Autodesk Fusion 360 part; units mm, degrees
(part 3 of 3)
sketch "M3 heat-set insert envelope sketch (1)" plane through (0, 0, 52) normal (0, 0, 1) x (1, 0, 0) in component "19 Rear M3 fastener envelopes TBD"
  circle A0 centre (-40, 90) radius 2.1
  dimension "d1035" = 40
  dimension "d1036" = 90
  dimension "d1037" = 2.1
  measures "d1035" horizontal distance of origin A0.centre
  measures "d1036" vertical distance of origin A0.centre
  measures "d1037" radius of A0
extrude "M3 heat-set insert envelope (1)" add sketch "M3 heat-set insert envelope sketch (1)" along normal blind 5 separate body makes body 40 in component "19 Rear M3 fastener envelopes TBD"
ref_plane "WorkPlane6" through (0, 0, 52) normal (0, 0, 1) x (1, 0, 0) in component "19 Rear M3 fastener envelopes TBD"
sketch "Insert thread clearance envelope sketch (1)" plane through (0, 0, 52) normal (0, 0, 1) x (1, 0, 0) in component "19 Rear M3 fastener envelopes TBD"
  circle A0 centre (-40, 90) radius 1.55
  dimension "d1042" = 40
  dimension "d1043" = 90
  dimension "d1044" = 1.55
  measures "d1042" horizontal distance of origin A0.centre
  measures "d1043" vertical distance of origin A0.centre
  measures "d1044" radius of A0
extrude "Insert thread clearance envelope (1)" cut sketch "Insert thread clearance envelope sketch (1)" along normal blind 5 bodies 40 in component "19 Rear M3 fastener envelopes TBD"
ref_plane "WorkPlane7" through (0, 0, 54.2) normal (0, 0, 1) x (1, 0, 0) in component "19 Rear M3 fastener envelopes TBD"
sketch "M3 screw shaft envelope sketch (1)" plane through (0, 0, 54.2) normal (0, 0, 1) x (1, 0, 0) in component "19 Rear M3 fastener envelopes TBD"
  circle A0 centre (-40, 90) radius 1.45
  dimension "d1049" = 40
  dimension "d1050" = 90
  dimension "d1051" = 1.45
  measures "d1049" horizontal distance of origin A0.centre
  measures "d1050" vertical distance of origin A0.centre
  measures "d1051" radius of A0
extrude "M3 screw shaft envelope (1)" add sketch "M3 screw shaft envelope sketch (1)" along normal blind 4 separate body makes body 41 in component "19 Rear M3 fastener envelopes TBD"
ref_plane "WorkPlane8" through (0, 0, 58.2) normal (0, 0, 1) x (1, 0, 0) in component "19 Rear M3 fastener envelopes TBD"
sketch "M3 low head envelope sketch (1)" plane through (0, 0, 58.2) normal (0, 0, 1) x (1, 0, 0) in component "19 Rear M3 fastener envelopes TBD"
  circle A0 centre (-40, 90) radius 2.75
  dimension "d1056" = 40
  dimension "d1057" = 90
  dimension "d1058" = 2.75
  measures "d1056" horizontal distance of origin A0.centre
  measures "d1057" vertical distance of origin A0.centre
  measures "d1058" radius of A0
extrude "M3 low head envelope (1)" add sketch "M3 low head envelope sketch (1)" along normal blind 1.8 separate body makes body 42 in component "19 Rear M3 fastener envelopes TBD"
ref_plane "WorkPlane10" through (0, 0, 58.2) normal (0, 0, 1) x (1, 0, 0) in component "02 Single rear cover"
sketch "M3 head recess sketch (2)" plane through (0, 0, 58.2) normal (0, 0, 1) x (1, 0, 0) in component "02 Single rear cover"
  circle A0 centre (-40, 172) radius 3
  dimension "d1063" = 40
  dimension "d1064" = 172
  dimension "d1065" = 3
  measures "d1063" horizontal distance of origin A0.centre
  measures "d1064" vertical distance of origin A0.centre
  measures "d1065" radius of A0
extrude "M3 head recess (2)" cut sketch "M3 head recess sketch (2)" along normal blind 1.9 bodies 2 in component "02 Single rear cover"
ref_plane "WorkPlane9" through (0, 0, 52) normal (0, 0, 1) x (1, 0, 0) in component "19 Rear M3 fastener envelopes TBD"
sketch "M3 heat-set insert envelope sketch (2)" plane through (0, 0, 52) normal (0, 0, 1) x (1, 0, 0) in component "19 Rear M3 fastener envelopes TBD"
  circle A0 centre (-40, 172) radius 2.1
  dimension "d1070" = 40
  dimension "d1071" = 172
  dimension "d1072" = 2.1
  measures "d1070" horizontal distance of origin A0.centre
  measures "d1071" vertical distance of origin A0.centre
  measures "d1072" radius of A0
extrude "M3 heat-set insert envelope (2)" add sketch "M3 heat-set insert envelope sketch (2)" along normal blind 5 separate body makes body 43 in component "19 Rear M3 fastener envelopes TBD"
ref_plane "WorkPlane10" through (0, 0, 52) normal (0, 0, 1) x (1, 0, 0) in component "19 Rear M3 fastener envelopes TBD"
sketch "Insert thread clearance envelope sketch (2)" plane through (0, 0, 52) normal (0, 0, 1) x (1, 0, 0) in component "19 Rear M3 fastener envelopes TBD"
  circle A0 centre (-40, 172) radius 1.55
  dimension "d1077" = 40
  dimension "d1078" = 172
  dimension "d1079" = 1.55
  measures "d1077" horizontal distance of origin A0.centre
  measures "d1078" vertical distance of origin A0.centre
  measures "d1079" radius of A0
extrude "Insert thread clearance envelope (2)" cut sketch "Insert thread clearance envelope sketch (2)" along normal blind 5 bodies 43 in component "19 Rear M3 fastener envelopes TBD"
ref_plane "WorkPlane11" through (0, 0, 54.2) normal (0, 0, 1) x (1, 0, 0) in component "19 Rear M3 fastener envelopes TBD"
sketch "M3 screw shaft envelope sketch (2)" plane through (0, 0, 54.2) normal (0, 0, 1) x (1, 0, 0) in component "19 Rear M3 fastener envelopes TBD"
  circle A0 centre (-40, 172) radius 1.45
  dimension "d1084" = 40
  dimension "d1085" = 172
  dimension "d1086" = 1.45
  measures "d1084" horizontal distance of origin A0.centre
  measures "d1085" vertical distance of origin A0.centre
  measures "d1086" radius of A0
extrude "M3 screw shaft envelope (2)" add sketch "M3 screw shaft envelope sketch (2)" along normal blind 4 separate body makes body 44 in component "19 Rear M3 fastener envelopes TBD"
ref_plane "WorkPlane12" through (0, 0, 58.2) normal (0, 0, 1) x (1, 0, 0) in component "19 Rear M3 fastener envelopes TBD"
sketch "M3 low head envelope sketch (2)" plane through (0, 0, 58.2) normal (0, 0, 1) x (1, 0, 0) in component "19 Rear M3 fastener envelopes TBD"
  circle A0 centre (-40, 172) radius 2.75
  dimension "d1091" = 40
  dimension "d1092" = 172
  dimension "d1093" = 2.75
  measures "d1091" horizontal distance of origin A0.centre
  measures "d1092" vertical distance of origin A0.centre
  measures "d1093" radius of A0
extrude "M3 low head envelope (2)" add sketch "M3 low head envelope sketch (2)" along normal blind 1.8 separate body makes body 45 in component "19 Rear M3 fastener envelopes TBD"
ref_plane "WorkPlane11" through (0, 0, 58.2) normal (0, 0, 1) x (1, 0, 0) in component "02 Single rear cover"
sketch "M3 head recess sketch (3)" plane through (0, 0, 58.2) normal (0, 0, 1) x (1, 0, 0) in component "02 Single rear cover"
  circle A0 centre (40, 8) radius 3
  dimension "d1098" = 40
  dimension "d1099" = 8
  dimension "d1100" = 3
  measures "d1098" horizontal distance of origin A0.centre
  measures "d1099" vertical distance of origin A0.centre
  measures "d1100" radius of A0
extrude "M3 head recess (3)" cut sketch "M3 head recess sketch (3)" along normal blind 1.9 bodies 2 in component "02 Single rear cover"
ref_plane "WorkPlane13" through (0, 0, 52) normal (0, 0, 1) x (1, 0, 0) in component "19 Rear M3 fastener envelopes TBD"
sketch "M3 heat-set insert envelope sketch (3)" plane through (0, 0, 52) normal (0, 0, 1) x (1, 0, 0) in component "19 Rear M3 fastener envelopes TBD"
  circle A0 centre (40, 8) radius 2.1
  dimension "d1105" = 40
  dimension "d1106" = 8
  dimension "d1107" = 2.1
  measures "d1105" horizontal distance of origin A0.centre
  measures "d1106" vertical distance of origin A0.centre
  measures "d1107" radius of A0
extrude "M3 heat-set insert envelope (3)" add sketch "M3 heat-set insert envelope sketch (3)" along normal blind 5 separate body makes body 46 in component "19 Rear M3 fastener envelopes TBD"
ref_plane "WorkPlane14" through (0, 0, 52) normal (0, 0, 1) x (1, 0, 0) in component "19 Rear M3 fastener envelopes TBD"
sketch "Insert thread clearance envelope sketch (3)" plane through (0, 0, 52) normal (0, 0, 1) x (1, 0, 0) in component "19 Rear M3 fastener envelopes TBD"
  circle A0 centre (40, 8) radius 1.55
  dimension "d1112" = 40
  dimension "d1113" = 8
  dimension "d1114" = 1.55
  measures "d1112" horizontal distance of origin A0.centre
  measures "d1113" vertical distance of origin A0.centre
  measures "d1114" radius of A0
extrude "Insert thread clearance envelope (3)" cut sketch "Insert thread clearance envelope sketch (3)" along normal blind 5 bodies 46 in component "19 Rear M3 fastener envelopes TBD"
ref_plane "WorkPlane15" through (0, 0, 54.2) normal (0, 0, 1) x (1, 0, 0) in component "19 Rear M3 fastener envelopes TBD"
sketch "M3 screw shaft envelope sketch (3)" plane through (0, 0, 54.2) normal (0, 0, 1) x (1, 0, 0) in component "19 Rear M3 fastener envelopes TBD"
  circle A0 centre (40, 8) radius 1.45
  dimension "d1119" = 40
  dimension "d1120" = 8
  dimension "d1121" = 1.45
  measures "d1119" horizontal distance of origin A0.centre
  measures "d1120" vertical distance of origin A0.centre
  measures "d1121" radius of A0
extrude "M3 screw shaft envelope (3)" add sketch "M3 screw shaft envelope sketch (3)" along normal blind 4 separate body makes body 47 in component "19 Rear M3 fastener envelopes TBD"
ref_plane "WorkPlane16" through (0, 0, 58.2) normal (0, 0, 1) x (1, 0, 0) in component "19 Rear M3 fastener envelopes TBD"
sketch "M3 low head envelope sketch (3)" plane through (0, 0, 58.2) normal (0, 0, 1) x (1, 0, 0) in component "19 Rear M3 fastener envelopes TBD"
  circle A0 centre (40, 8) radius 2.75
  dimension "d1126" = 40
  dimension "d1127" = 8
  dimension "d1128" = 2.75
  measures "d1126" horizontal distance of origin A0.centre
  measures "d1127" vertical distance of origin A0.centre
  measures "d1128" radius of A0
extrude "M3 low head envelope (3)" add sketch "M3 low head envelope sketch (3)" along normal blind 1.8 separate body makes body 48 in component "19 Rear M3 fastener envelopes TBD"
ref_plane "WorkPlane12" through (0, 0, 58.2) normal (0, 0, 1) x (1, 0, 0) in component "02 Single rear cover"
sketch "M3 head recess sketch (4)" plane through (0, 0, 58.2) normal (0, 0, 1) x (1, 0, 0) in component "02 Single rear cover"
  circle A0 centre (40, 90) radius 3
  dimension "d1133" = 40
  dimension "d1134" = 90
  dimension "d1135" = 3
  measures "d1133" horizontal distance of origin A0.centre
  measures "d1134" vertical distance of origin A0.centre
  measures "d1135" radius of A0
extrude "M3 head recess (4)" cut sketch "M3 head recess sketch (4)" along normal blind 1.9 bodies 2 in component "02 Single rear cover"
ref_plane "WorkPlane17" through (0, 0, 52) normal (0, 0, 1) x (1, 0, 0) in component "19 Rear M3 fastener envelopes TBD"
sketch "M3 heat-set insert envelope sketch (4)" plane through (0, 0, 52) normal (0, 0, 1) x (1, 0, 0) in component "19 Rear M3 fastener envelopes TBD"
  circle A0 centre (40, 90) radius 2.1
  dimension "d1140" = 40
  dimension "d1141" = 90
  dimension "d1142" = 2.1
  measures "d1140" horizontal distance of origin A0.centre
  measures "d1141" vertical distance of origin A0.centre
  measures "d1142" radius of A0
extrude "M3 heat-set insert envelope (4)" add sketch "M3 heat-set insert envelope sketch (4)" along normal blind 5 separate body makes body 49 in component "19 Rear M3 fastener envelopes TBD"
ref_plane "WorkPlane18" through (0, 0, 52) normal (0, 0, 1) x (1, 0, 0) in component "19 Rear M3 fastener envelopes TBD"
sketch "Insert thread clearance envelope sketch (4)" plane through (0, 0, 52) normal (0, 0, 1) x (1, 0, 0) in component "19 Rear M3 fastener envelopes TBD"
  circle A0 centre (40, 90) radius 1.55
  dimension "d1147" = 40
  dimension "d1148" = 90
  dimension "d1149" = 1.55
  measures "d1147" horizontal distance of origin A0.centre
  measures "d1148" vertical distance of origin A0.centre
  measures "d1149" radius of A0
extrude "Insert thread clearance envelope (4)" cut sketch "Insert thread clearance envelope sketch (4)" along normal blind 5 bodies 49 in component "19 Rear M3 fastener envelopes TBD"
ref_plane "WorkPlane19" through (0, 0, 54.2) normal (0, 0, 1) x (1, 0, 0) in component "19 Rear M3 fastener envelopes TBD"
sketch "M3 screw shaft envelope sketch (4)" plane through (0, 0, 54.2) normal (0, 0, 1) x (1, 0, 0) in component "19 Rear M3 fastener envelopes TBD"
  circle A0 centre (40, 90) radius 1.45
  dimension "d1154" = 40
  dimension "d1155" = 90
  dimension "d1156" = 1.45
  measures "d1154" horizontal distance of origin A0.centre
  measures "d1155" vertical distance of origin A0.centre
  measures "d1156" radius of A0
extrude "M3 screw shaft envelope (4)" add sketch "M3 screw shaft envelope sketch (4)" along normal blind 4 separate body makes body 50 in component "19 Rear M3 fastener envelopes TBD"
ref_plane "WorkPlane20" through (0, 0, 58.2) normal (0, 0, 1) x (1, 0, 0) in component "19 Rear M3 fastener envelopes TBD"
sketch "M3 low head envelope sketch (4)" plane through (0, 0, 58.2) normal (0, 0, 1) x (1, 0, 0) in component "19 Rear M3 fastener envelopes TBD"
  circle A0 centre (40, 90) radius 2.75
  dimension "d1161" = 40
  dimension "d1162" = 90
  dimension "d1163" = 2.75
  measures "d1161" horizontal distance of origin A0.centre
  measures "d1162" vertical distance of origin A0.centre
  measures "d1163" radius of A0
extrude "M3 low head envelope (4)" add sketch "M3 low head envelope sketch (4)" along normal blind 1.8 separate body makes body 51 in component "19 Rear M3 fastener envelopes TBD"
ref_plane "WorkPlane13" through (0, 0, 58.2) normal (0, 0, 1) x (1, 0, 0) in component "02 Single rear cover"
sketch "M3 head recess sketch (5)" plane through (0, 0, 58.2) normal (0, 0, 1) x (1, 0, 0) in component "02 Single rear cover"
  circle A0 centre (40, 172) radius 3
  dimension "d1168" = 40
  dimension "d1169" = 172
  dimension "d1170" = 3
  measures "d1168" horizontal distance of origin A0.centre
  measures "d1169" vertical distance of origin A0.centre
  measures "d1170" radius of A0
extrude "M3 head recess (5)" cut sketch "M3 head recess sketch (5)" along normal blind 1.9 bodies 2 in component "02 Single rear cover"
ref_plane "WorkPlane21" through (0, 0, 52) normal (0, 0, 1) x (1, 0, 0) in component "19 Rear M3 fastener envelopes TBD"
sketch "M3 heat-set insert envelope sketch (5)" plane through (0, 0, 52) normal (0, 0, 1) x (1, 0, 0) in component "19 Rear M3 fastener envelopes TBD"
  circle A0 centre (40, 172) radius 2.1
  dimension "d1175" = 40
  dimension "d1176" = 172
  dimension "d1177" = 2.1
  measures "d1175" horizontal distance of origin A0.centre
  measures "d1176" vertical distance of origin A0.centre
  measures "d1177" radius of A0
extrude "M3 heat-set insert envelope (5)" add sketch "M3 heat-set insert envelope sketch (5)" along normal blind 5 separate body makes body 52 in component "19 Rear M3 fastener envelopes TBD"
ref_plane "WorkPlane22" through (0, 0, 52) normal (0, 0, 1) x (1, 0, 0) in component "19 Rear M3 fastener envelopes TBD"
sketch "Insert thread clearance envelope sketch (5)" plane through (0, 0, 52) normal (0, 0, 1) x (1, 0, 0) in component "19 Rear M3 fastener envelopes TBD"
  circle A0 centre (40, 172) radius 1.55
  dimension "d1182" = 40
  dimension "d1183" = 172
  dimension "d1184" = 1.55
  measures "d1182" horizontal distance of origin A0.centre
  measures "d1183" vertical distance of origin A0.centre
  measures "d1184" radius of A0
extrude "Insert thread clearance envelope (5)" cut sketch "Insert thread clearance envelope sketch (5)" along normal blind 5 bodies 52 in component "19 Rear M3 fastener envelopes TBD"
ref_plane "WorkPlane23" through (0, 0, 54.2) normal (0, 0, 1) x (1, 0, 0) in component "19 Rear M3 fastener envelopes TBD"
sketch "M3 screw shaft envelope sketch (5)" plane through (0, 0, 54.2) normal (0, 0, 1) x (1, 0, 0) in component "19 Rear M3 fastener envelopes TBD"
  circle A0 centre (40, 172) radius 1.45
  dimension "d1189" = 40
  dimension "d1190" = 172
  dimension "d1191" = 1.45
  measures "d1189" horizontal distance of origin A0.centre
  measures "d1190" vertical distance of origin A0.centre
  measures "d1191" radius of A0
extrude "M3 screw shaft envelope (5)" add sketch "M3 screw shaft envelope sketch (5)" along normal blind 4 separate body makes body 53 in component "19 Rear M3 fastener envelopes TBD"
ref_plane "WorkPlane24" through (0, 0, 58.2) normal (0, 0, 1) x (1, 0, 0) in component "19 Rear M3 fastener envelopes TBD"
sketch "M3 low head envelope sketch (5)" plane through (0, 0, 58.2) normal (0, 0, 1) x (1, 0, 0) in component "19 Rear M3 fastener envelopes TBD"
  circle A0 centre (40, 172) radius 2.75
  dimension "d1196" = 40
  dimension "d1197" = 172
  dimension "d1198" = 2.75
  measures "d1196" horizontal distance of origin A0.centre
  measures "d1197" vertical distance of origin A0.centre
  measures "d1198" radius of A0
extrude "M3 low head envelope (5)" add sketch "M3 low head envelope sketch (5)" along normal blind 1.8 separate body makes body 54 in component "19 Rear M3 fastener envelopes TBD"
component "01 Main housing" placed x (1, 0, 0) y (0, 1, 0) z (0, 0, 1) at (0, 0, 0)
component "02 Single rear cover" placed x (1, 0, 0) y (0, 1, 0) z (0, 0, 1) at (0, 0, 0)
component "03 Removable sampling chamber" placed x (1, 0, 0) y (0, 1, 0) z (0, 0, 1) at (0, 0, 0)
component "04 Internal chamber lid" placed x (1, 0, 0) y (0, 1, 0) z (0, 0, 1) at (0, 0, 0)
component "05 Feedthrough seal envelope TBD" placed x (1, 0, 0) y (0, 1, 0) z (0, 0, 1) at (0, 0, 0)
component "06 Gas fitting envelopes TBD" placed x (1, 0, 0) y (0, 1, 0) z (0, 0, 1) at (0, 0, 0)
component "07 Guition 4.3in envelope — depth TBD" placed x (1, 0, 0) y (0, 1, 0) z (0, 0, 1) at (0, 0, 0)
component "08 Active display reference" placed x (1, 0, 0) y (0, 1, 0) z (0, 0, 1) at (0, 0, 0)
component "09 Removable electronics carrier" placed x (1, 0, 0) y (0, 1, 0) z (0, 0, 1) at (0, 0, 0)
component "10 Future PCB and component envelope TBD" placed x (1, 0, 0) y (0, 1, 0) z (0, 0, 1) at (0, 0, 0)
component "11 Protected FMA holder envelope TBD" placed x (1, 0, 0) y (0, 1, 0) z (0, 0, 1) at (0, 0, 0)
component "12 Two 18650 cell envelopes" placed x (1, 0, 0) y (0, 1, 0) z (0, 0, 1) at (0, 0, 0)
component "13 Battery plug and cable clearance TBD" placed x (1, 0, 0) y (0, 1, 0) z (0, 0, 1) at (0, 0, 0)
component "14 Supported USB-C mounting insert TBD" placed x (1, 0, 0) y (0, 1, 0) z (0, 0, 1) at (0, 0, 0)
component "15 USB daughterboard envelope 0.60mm" placed x (1, 0, 0) y (0, 1, 0) z (0, 0, 1) at (0, 0, 0)
component "16 Right momentary button envelope TBD" placed x (1, 0, 0) y (0, 1, 0) z (0, 0, 1) at (0, 0, 0)
component "18 Wiring route clearance envelopes" placed x (1, 0, 0) y (0, 1, 0) z (0, 0, 1) at (0, 0, 0)
component "17 Chamber sensor envelopes TBD" placed x (1, 0, 0) y (0, 1, 0) z (0, 0, 1) at (0, 0, 0)
component "19 Rear M3 fastener envelopes TBD" placed x (1, 0, 0) y (0, 1, 0) z (0, 0, 1) at (0, 0, 0)
equation "CaseWidth = 95 mm" comment "Provisional outer width"
equation "CaseHeight = 180 mm" comment "Provisional outer height"
equation "CaseDepth = 60 mm" comment "Provisional total depth including rear cover"
equation "Wall = 3 mm" comment "Initial PLA shell wall"
equation "Cover = 3 mm" comment "Single rear cover thickness"
equation "CornerRadius = 8 mm" comment "Outside corner radius"
equation "CoverGap = 0.25 mm" comment "Provisional cover seating clearance"
equation "DisplayWidth = 69.41 mm" comment "Verified conservative Guition module outline"
equation "DisplayHeight = 117.01 mm" comment "Verified conservative Guition module outline"
equation "DisplayDepth = 13.8 mm" comment "PROVISIONAL: shell-variant depth; confirm purchased unit"
equation "DisplayBottom = 10 mm" comment "Module lower edge"
equation "ActiveWidth = 56.16 mm" comment "Verified active display width"
equation "ActiveHeight = 93.60 mm" comment "Verified active display height"
equation "WindowMargin = 0.5 mm" comment "Provisional margin around active area"
equation "BossInset = 7.5 mm" comment "Rear-cover screw centre inset from left/right"
equation "BossRadius = 4.5 mm" comment "Cover screw boss outer radius"
equation "InsertRadius = 2.1 mm" comment "PROVISIONAL M3 insert pilot radius; fit coupon required"
equation "InsertDepth = 5 mm" comment "PROVISIONAL M3 insert length"
equation "ScrewClearance = 1.7 mm" comment "M3 rear-cover clearance radius"
equation "ChamberWidth = 70 mm" comment "Removable chamber outside width"
equation "ChamberHeight = 43 mm" comment "Removable chamber outside height"
equation "ChamberTopGap = 5 mm" comment "Clearance to case top"
equation "ChamberBottom = CaseHeight - ChamberTopGap - ChamberHeight" comment "Derived chamber lower edge"
equation "ChamberFront = 3.5 mm" comment "Chamber front wall position"
equation "ChamberWall = 2 mm" comment "Concept chamber wall; seal details pending"
equation "ChamberLid = 2 mm" comment "Internally accessible chamber lid"
equation "ChamberRear = CaseDepth - Cover - 0.5 mm" comment "Rear of closed chamber"
equation "GasY = ChamberBottom + ChamberHeight / 2" comment "Gas inlet/outlet elevation"
equation "GasZ = 12 mm" comment "Gas path centre depth"
equation "GasBoreRadius = 2.5 mm" comment "5 mm nominal tube ID"
equation "GasPassRadius = 4.5 mm" comment "PROVISIONAL housing clearance for side fitting"
equation "UsbY = 68 mm" comment "Left charging connector centre height"
equation "UsbZ = 34 mm" comment "USB connector depth centre"
equation "ButtonY = 102 mm" comment "Right-side power button centre height"
equation "ButtonZ = 42 mm" comment "Button depth centre"
equation "ButtonRadius = 6 mm" comment "Owned nominal 12 mm mounting diameter; confirm"
equation "d42 = -( -CaseWidth / 2 )"
equation "d43 = CaseWidth"
equation "d44 = CaseHeight"
equation "d45 = CaseDepth - Cover"
equation "d48 = CornerRadius"
equation "d49 = Wall"
equation "d51 = -( -CaseWidth / 2 + Wall )"
equation "d52 = Wall"
equation "d53 = CaseWidth - 2 * Wall"
equation "d54 = CaseHeight - 2 * Wall"
equation "d55 = CaseDepth"
equation "d58 = CornerRadius - Wall"
equation "d61 = -( -( ActiveWidth + 2 * WindowMargin ) / 2 )"
equation "d62 = DisplayBottom + ( DisplayHeight - ActiveHeight ) / 2 - WindowMargin"
equation "d63 = ActiveWidth + 2 * WindowMargin"
equation "d64 = ActiveHeight + 2 * WindowMargin"
equation "d65 = Wall + 2 mm"
equation "d67 = Wall"
equation "d69 = -( -CaseWidth / 2 + BossInset )"
equation "d71 = BossRadius"
equation "d72 = CaseDepth - Cover - Wall"
equation "d74 = Wall"
equation "d76 = -( -CaseWidth / 2 + Wall )"
equation "d77 = ( 8 mm ) - BossRadius"
equation "d78 = BossInset - Wall"
equation "d79 = 2 * BossRadius"
equation "d80 = CaseDepth - Cover - Wall"
equation "d82 = CaseDepth - Cover - InsertDepth"
equation "d84 = -( -CaseWidth / 2 + BossInset )"
equation "d86 = InsertRadius"
equation "d87 = InsertDepth + 0.1 mm"
equation "d89 = Wall"
equation "d91 = -( -CaseWidth / 2 + BossInset )"
equation "d92 = CaseHeight / 2"
equation "d93 = BossRadius"
equation "d94 = CaseDepth - Cover - Wall"
equation "d96 = Wall"
equation "d98 = -( -CaseWidth / 2 + Wall )"
equation "d99 = ( CaseHeight / 2 ) - BossRadius"
equation "d100 = BossInset - Wall"
equation "d101 = 2 * BossRadius"
equation "d102 = CaseDepth - Cover - Wall"
equation "d104 = CaseDepth - Cover - InsertDepth"
equation "d106 = -( -CaseWidth / 2 + BossInset )"
equation "d107 = CaseHeight / 2"
equation "d108 = InsertRadius"
equation "d109 = InsertDepth + 0.1 mm"
equation "d111 = Wall"
equation "d113 = -( -CaseWidth / 2 + BossInset )"
equation "d114 = CaseHeight - 8 mm"
equation "d115 = BossRadius"
equation "d116 = CaseDepth - Cover - Wall"
equation "d118 = Wall"
equation "d120 = -( -CaseWidth / 2 + Wall )"
equation "d121 = ( CaseHeight - 8 mm ) - BossRadius"
equation "d122 = BossInset - Wall"
equation "d123 = 2 * BossRadius"
equation "d124 = CaseDepth - Cover - Wall"
equation "d126 = CaseDepth - Cover - InsertDepth"
equation "d128 = -( -CaseWidth / 2 + BossInset )"
equation "d129 = CaseHeight - 8 mm"
equation "d130 = InsertRadius"
equation "d131 = InsertDepth + 0.1 mm"
equation "d133 = Wall"
equation "d135 = CaseWidth / 2 - BossInset"
equation "d137 = BossRadius"
equation "d138 = CaseDepth - Cover - Wall"
equation "d140 = Wall"
equation "d142 = CaseWidth / 2 - BossInset"
equation "d143 = ( 8 mm ) - BossRadius"
equation "d144 = BossInset - Wall"
equation "d145 = 2 * BossRadius"
equation "d146 = CaseDepth - Cover - Wall"
equation "d148 = CaseDepth - Cover - InsertDepth"
equation "d150 = CaseWidth / 2 - BossInset"
equation "d152 = InsertRadius"
equation "d153 = InsertDepth + 0.1 mm"
equation "d155 = Wall"
equation "d157 = CaseWidth / 2 - BossInset"
equation "d158 = CaseHeight / 2"
equation "d159 = BossRadius"
equation "d160 = CaseDepth - Cover - Wall"
equation "d162 = Wall"
equation "d164 = CaseWidth / 2 - BossInset"
equation "d165 = ( CaseHeight / 2 ) - BossRadius"
equation "d166 = BossInset - Wall"
equation "d167 = 2 * BossRadius"
equation "d168 = CaseDepth - Cover - Wall"
equation "d170 = CaseDepth - Cover - InsertDepth"
equation "d172 = CaseWidth / 2 - BossInset"
equation "d173 = CaseHeight / 2"
equation "d174 = InsertRadius"
equation "d175 = InsertDepth + 0.1 mm"
equation "d177 = Wall"
equation "d179 = CaseWidth / 2 - BossInset"
equation "d180 = CaseHeight - 8 mm"
equation "d181 = BossRadius"
equation "d182 = CaseDepth - Cover - Wall"
equation "d184 = Wall"
equation "d186 = CaseWidth / 2 - BossInset"
equation "d187 = ( CaseHeight - 8 mm ) - BossRadius"
equation "d188 = BossInset - Wall"
equation "d189 = 2 * BossRadius"
equation "d190 = CaseDepth - Cover - Wall"
equation "d192 = CaseDepth - Cover - InsertDepth"
equation "d194 = CaseWidth / 2 - BossInset"
equation "d195 = CaseHeight - 8 mm"
equation "d196 = InsertRadius"
equation "d197 = InsertDepth + 0.1 mm"
equation "d199 = -CaseWidth / 2 - 1 mm"
equation "d201 = -( -( GasZ ) )"
equation "d202 = GasY"
equation "d203 = GasPassRadius"
equation "d204 = CaseWidth + 2 mm"
equation "d206 = -CaseWidth / 2 - 1 mm"
equation "d208 = -( -( ButtonZ ) )"
equation "d209 = ButtonY"
equation "d210 = ButtonRadius"
equation "d211 = Wall + 2 mm"
equation "d213 = CaseWidth / 2 - Wall - 1 mm"
equation "d215 = -( -( ( UsbZ - 8 mm ) + ( 16 mm ) ) )"
equation "d216 = UsbY - 10 mm"
equation "d219 = Wall + 2 mm"
equation "d221 = CaseDepth - Cover + CoverGap"
equation "d223 = -( -CaseWidth / 2 )"
equation "d224 = CaseWidth"
equation "d225 = CaseHeight"
equation "d226 = Cover - CoverGap"
equation "d229 = CornerRadius"
equation "d230 = CaseDepth - Cover"
equation "d232 = -( -CaseWidth / 2 + BossInset )"
equation "d234 = ScrewClearance"
equation "d235 = Cover + 1 mm"
equation "d237 = CaseDepth - Cover"
equation "d239 = -( -CaseWidth / 2 + BossInset )"
equation "d240 = CaseHeight / 2"
equation "d241 = ScrewClearance"
equation "d242 = Cover + 1 mm"
equation "d244 = CaseDepth - Cover"
equation "d246 = -( -CaseWidth / 2 + BossInset )"
equation "d247 = CaseHeight - 8 mm"
equation "d248 = ScrewClearance"
equation "d249 = Cover + 1 mm"
equation "d251 = CaseDepth - Cover"
equation "d253 = CaseWidth / 2 - BossInset"
equation "d255 = ScrewClearance"
equation "d256 = Cover + 1 mm"
equation "d258 = CaseDepth - Cover"
equation "d260 = CaseWidth / 2 - BossInset"
equation "d261 = CaseHeight / 2"
equation "d262 = ScrewClearance"
equation "d263 = Cover + 1 mm"
equation "d265 = CaseDepth - Cover"
equation "d267 = CaseWidth / 2 - BossInset"
equation "d268 = CaseHeight - 8 mm"
equation "d269 = ScrewClearance"
equation "d270 = Cover + 1 mm"
equation "d272 = ChamberFront"
equation "d274 = -( -ChamberWidth / 2 )"
equation "d275 = ChamberBottom"
equation "d276 = ChamberWidth"
equation "d277 = ChamberHeight"
equation "d278 = ChamberRear - ChamberFront - ChamberLid"
equation "d280 = ChamberFront + ChamberWall"
equation "d282 = -( -ChamberWidth / 2 + ChamberWall )"
equation "d283 = ChamberBottom + ChamberWall"
equation "d284 = ChamberWidth - 2 * ChamberWall"
equation "d285 = ChamberHeight - 2 * ChamberWall"
equation "d286 = ChamberRear - ChamberFront"
equation "d288 = -ChamberWidth / 2 - 1 mm"
equation "d290 = -( -( GasZ ) )"
equation "d291 = GasY"
equation "d293 = ChamberWidth + 2 mm"
equation "d295 = ChamberFront + ChamberWall"
equation "d297 = -( -ChamberWidth / 2 + 5 mm )"
equation "d298 = ChamberBottom + 4 mm"
equation "d300 = ChamberRear - ChamberLid - ChamberFront - ChamberWall"
equation "d302 = ChamberRear - ChamberLid - 4 mm"
equation "d304 = -( -ChamberWidth / 2 + 5 mm )"
equation "d305 = ChamberBottom + 4 mm"
equation "d309 = ChamberFront + ChamberWall"
equation "d311 = -( -ChamberWidth / 2 + 5 mm )"
equation "d312 = ChamberBottom + ChamberHeight - 4 mm"
equation "d314 = ChamberRear - ChamberLid - ChamberFront - ChamberWall"
equation "d316 = ChamberRear - ChamberLid - 4 mm"
equation "d318 = -( -ChamberWidth / 2 + 5 mm )"
equation "d319 = ChamberBottom + ChamberHeight - 4 mm"
equation "d323 = ChamberFront + ChamberWall"
equation "d325 = ChamberWidth / 2 - 5 mm"
equation "d326 = ChamberBottom + 4 mm"
equation "d328 = ChamberRear - ChamberLid - ChamberFront - ChamberWall"
equation "d330 = ChamberRear - ChamberLid - 4 mm"
equation "d332 = ChamberWidth / 2 - 5 mm"
equation "d333 = ChamberBottom + 4 mm"
equation "d337 = ChamberFront + ChamberWall"
equation "d339 = ChamberWidth / 2 - 5 mm"
equation "d340 = ChamberBottom + ChamberHeight - 4 mm"
equation "d342 = ChamberRear - ChamberLid - ChamberFront - ChamberWall"
equation "d344 = ChamberRear - ChamberLid - 4 mm"
equation "d346 = ChamberWidth / 2 - 5 mm"
equation "d347 = ChamberBottom + ChamberHeight - 4 mm"
equation "d353 = -( -ChamberWidth / 2 - 6 mm )"
equation "d354 = ( ChamberBottom + 5 mm ) - 3 mm"
equation "d361 = -( -ChamberWidth / 2 - 3 mm )"
equation "d362 = ChamberBottom + 5 mm"
equation "d366 = Wall"
equation "d368 = -( -ChamberWidth / 2 - 3 mm )"
equation "d369 = ChamberBottom + 5 mm"
equation "d371 = 47 mm - Wall"
equation "d375 = -( -ChamberWidth / 2 - 3 mm )"
equation "d376 = ChamberBottom + 5 mm"
equation "d382 = -( -ChamberWidth / 2 - 6 mm )"
equation "d383 = ( ChamberBottom + ChamberHeight - 12 mm ) - 3 mm"
equation "d390 = -( -ChamberWidth / 2 - 3 mm )"
equation "d391 = ChamberBottom + ChamberHeight - 12 mm"
equation "d395 = Wall"
equation "d397 = -( -ChamberWidth / 2 - 3 mm )"
equation "d398 = ChamberBottom + ChamberHeight - 12 mm"
equation "d400 = 47 mm - Wall"
equation "d404 = -( -ChamberWidth / 2 - 3 mm )"
equation "d405 = ChamberBottom + ChamberHeight - 12 mm"
equation "d411 = ChamberWidth / 2 - 0.5 mm"
equation "d412 = ( ChamberBottom + 5 mm ) - 3 mm"
equation "d419 = ChamberWidth / 2 + 3 mm"
equation "d420 = ChamberBottom + 5 mm"
equation "d424 = Wall"
equation "d426 = ChamberWidth / 2 + 3 mm"
equation "d427 = ChamberBottom + 5 mm"
equation "d429 = 47 mm - Wall"
equation "d433 = ChamberWidth / 2 + 3 mm"
equation "d434 = ChamberBottom + 5 mm"
equation "d440 = ChamberWidth / 2 - 0.5 mm"
equation "d441 = ( ChamberBottom + ChamberHeight - 12 mm ) - 3 mm"
equation "d448 = ChamberWidth / 2 + 3 mm"
equation "d449 = ChamberBottom + ChamberHeight - 12 mm"
equation "d453 = Wall"
equation "d455 = ChamberWidth / 2 + 3 mm"
equation "d456 = ChamberBottom + ChamberHeight - 12 mm"
equation "d458 = 47 mm - Wall"
equation "d462 = ChamberWidth / 2 + 3 mm"
equation "d463 = ChamberBottom + ChamberHeight - 12 mm"
equation "d467 = ChamberRear - ChamberLid"
equation "d469 = -( -ChamberWidth / 2 )"
equation "d470 = ChamberBottom"
equation "d471 = ChamberWidth"
equation "d472 = ChamberHeight"
equation "d473 = ChamberLid"
equation "d475 = ChamberRear - ChamberLid - 0.1 mm"
equation "d477 = -( -ChamberWidth / 2 + 5 mm )"
equation "d478 = ChamberBottom + 4 mm"
equation "d480 = ChamberLid + 0.2 mm"
equation "d482 = ChamberRear - ChamberLid - 0.1 mm"
equation "d484 = -( -ChamberWidth / 2 + 5 mm )"
equation "d485 = ChamberBottom + ChamberHeight - 4 mm"
equation "d487 = ChamberLid + 0.2 mm"
equation "d489 = ChamberRear - ChamberLid - 0.1 mm"
equation "d491 = ChamberWidth / 2 - 5 mm"
equation "d492 = ChamberBottom + 4 mm"
equation "d494 = ChamberLid + 0.2 mm"
equation "d496 = ChamberRear - ChamberLid - 0.1 mm"
equation "d498 = ChamberWidth / 2 - 5 mm"
equation "d499 = ChamberBottom + ChamberHeight - 4 mm"
equation "d501 = ChamberLid + 0.2 mm"
equation "d503 = ChamberBottom - 0.1 mm"
equation "d505 = -( -5 mm )"
equation "d506 = -( -( ( 48 mm ) + ( 5 mm ) ) )"
equation "d509 = ChamberWall + 0.2 mm"
equation "d513 = -( -5 mm )"
equation "d514 = ChamberBottom"
equation "d516 = ChamberWall"
equation "d519 = -CaseWidth / 2 - 6 mm"
equation "d521 = -( -( GasZ ) )"
equation "d522 = GasY"
equation "d524 = CaseWidth / 2 + 6 mm - ChamberWidth / 2 + ChamberWall"
equation "d526 = -CaseWidth / 2 - 6 mm"
equation "d528 = -( -( GasZ ) )"
equation "d529 = GasY"
equation "d530 = GasBoreRadius"
equation "d531 = CaseWidth / 2 + 6 mm - ChamberWidth / 2 + ChamberWall"
equation "d533 = ChamberWidth / 2 - ChamberWall"
equation "d535 = -( -( GasZ ) )"
equation "d536 = GasY"
equation "d538 = CaseWidth / 2 + 6 mm - ChamberWidth / 2 + ChamberWall"
equation "d540 = ChamberWidth / 2 - ChamberWall"
equation "d542 = -( -( GasZ ) )"
equation "d543 = GasY"
equation "d544 = GasBoreRadius"
equation "d545 = CaseWidth / 2 + 6 mm - ChamberWidth / 2 + ChamberWall"
equation "d547 = Wall + 0.3 mm"
equation "d549 = -( -DisplayWidth / 2 )"
equation "d550 = DisplayBottom"
equation "d551 = DisplayWidth"
equation "d552 = DisplayHeight"
equation "d553 = DisplayDepth"
equation "d555 = Wall + 0.2 mm"
equation "d557 = -( -ActiveWidth / 2 )"
equation "d558 = DisplayBottom + ( DisplayHeight - ActiveHeight ) / 2"
equation "d559 = ActiveWidth"
equation "d560 = ActiveHeight"
equation "d565 = -( -35 mm )"
equation "d581 = -( -35 mm )"
equation "d589 = -( -35 mm )"
equation "d597 = -( -41 mm )"
equation "d598 = ( 20 mm ) - 3 mm"
equation "d605 = -( -38 mm )"
equation "d610 = Wall"
equation "d612 = -( -38 mm )"
equation "d615 = 19 mm - Wall"
equation "d619 = -( -38 mm )"
equation "d621 = InsertRadius"
equation "d626 = -( -41 mm )"
equation "d627 = ( 124 mm ) - 3 mm"
equation "d634 = -( -38 mm )"
equation "d639 = Wall"
equation "d641 = -( -38 mm )"
equation "d644 = 19 mm - Wall"
equation "d648 = -( -38 mm )"
equation "d650 = InsertRadius"
equation "d656 = ( 20 mm ) - 3 mm"
equation "d668 = Wall"
equation "d673 = 19 mm - Wall"
equation "d679 = InsertRadius"
equation "d685 = ( 124 mm ) - 3 mm"
equation "d697 = Wall"
equation "d702 = 19 mm - Wall"
equation "d708 = InsertRadius"
equation "d713 = -( -32 mm )"
equation "d721 = -( -27 mm )"
equation "d729 = -( -27 mm )"
equation "d737 = -( -22 mm )"
equation "d745 = -( -20 mm )"
equation "d753 = -( -10 mm )"
equation "d754 = -( -( 39 mm ) )"
equation "d761 = -( -( 39 mm ) )"
equation "d773 = CaseWidth / 2 - Wall"
equation "d775 = -( -( ( UsbZ - 7.75 mm ) + ( 15.5 mm ) ) )"
equation "d776 = UsbY - 9.75 mm"
equation "d779 = Wall"
equation "d781 = CaseWidth / 2 - Wall - 2 mm"
equation "d783 = -( -( ( UsbZ - 10 mm ) + ( 20 mm ) ) )"
equation "d784 = UsbY - 12 mm"
equation "d789 = CaseWidth / 2 - Wall - 2.1 mm"
equation "d791 = -( -( ( UsbZ - 1.93 mm ) + ( 3.86 mm ) ) )"
equation "d792 = UsbY - 4.82 mm"
equation "d795 = Wall + 2.2 mm"
equation "d797 = CaseWidth / 2 - Wall - 2.1 mm"
equation "d799 = -( -( ( UsbZ - 1.93 mm ) + ( 3.86 mm ) ) )"
equation "d800 = UsbY - 4.82 mm"
equation "d805 = UsbZ - 0.3 mm"
equation "d808 = UsbY - 8 mm"
equation "d813 = UsbZ - 1.5 mm"
equation "d816 = UsbY - 4.5 mm"
equation "d817 = CaseWidth / 2 - 34 mm"
equation "d821 = UsbZ - 2.3 mm"
equation "d824 = UsbY - 8 mm"
equation "d825 = CaseWidth / 2 - Wall - 2 mm - 29 mm"
equation "d829 = UsbZ - 2.3 mm"
equation "d832 = UsbY + 6 mm"
equation "d833 = CaseWidth / 2 - Wall - 2 mm - 29 mm"
equation "d837 = -CaseWidth / 2"
equation "d839 = -( -( ButtonZ ) )"
equation "d840 = ButtonY"
equation "d844 = -CaseWidth / 2 - 1.5 mm"
equation "d846 = -( -( ButtonZ ) )"
equation "d847 = ButtonY"
equation "d851 = -CaseWidth / 2 + 18 mm"
equation "d853 = -( -( ( ButtonZ - 6 mm ) + ( 12 mm ) ) )"
equation "d854 = ButtonY - 6 mm"
equation "d915 = -( -5 mm )"
equation "d929 = UsbZ - 0.4 mm"
equation "d932 = UsbY - 4.6 mm"
equation "d940 = GasY"
equation "d947 = GasY"
equation "d954 = GasY - 5 mm"
equation "d961 = -( -32.4 mm )"
equation "d962 = ChamberBottom + 13 mm"
equation "d969 = -( -26 mm )"
equation "d970 = ChamberBottom + 3 mm"
equation "d977 = -( -26 mm )"
equation "d978 = ChamberBottom + 3 mm"
equation "d986 = GasY - 8.5 mm"
equation "d991 = CaseDepth - 1.8 mm"
equation "d993 = -( -CaseWidth / 2 + BossInset )"
equation "d998 = CaseDepth - Cover - InsertDepth"
equation "d1000 = -( -CaseWidth / 2 + BossInset )"
equation "d1002 = InsertRadius"
equation "d1003 = InsertDepth"
equation "d1005 = CaseDepth - Cover - InsertDepth"
equation "d1007 = -( -CaseWidth / 2 + BossInset )"
equation "d1010 = InsertDepth"
equation "d1012 = CaseDepth - 5.8 mm"
equation "d1014 = -( -CaseWidth / 2 + BossInset )"
equation "d1019 = CaseDepth - 1.8 mm"
equation "d1021 = -( -CaseWidth / 2 + BossInset )"
equation "d1026 = CaseDepth - 1.8 mm"
equation "d1028 = -( -CaseWidth / 2 + BossInset )"
equation "d1029 = CaseHeight / 2"
equation "d1033 = CaseDepth - Cover - InsertDepth"
equation "d1035 = -( -CaseWidth / 2 + BossInset )"
equation "d1036 = CaseHeight / 2"
equation "d1037 = InsertRadius"
equation "d1038 = InsertDepth"
equation "d1040 = CaseDepth - Cover - InsertDepth"
equation "d1042 = -( -CaseWidth / 2 + BossInset )"
equation "d1043 = CaseHeight / 2"
equation "d1045 = InsertDepth"
equation "d1047 = CaseDepth - 5.8 mm"
equation "d1049 = -( -CaseWidth / 2 + BossInset )"
equation "d1050 = CaseHeight / 2"
equation "d1054 = CaseDepth - 1.8 mm"
equation "d1056 = -( -CaseWidth / 2 + BossInset )"
equation "d1057 = CaseHeight / 2"
equation "d1061 = CaseDepth - 1.8 mm"
equation "d1063 = -( -CaseWidth / 2 + BossInset )"
equation "d1064 = CaseHeight - 8 mm"
equation "d1068 = CaseDepth - Cover - InsertDepth"
equation "d1070 = -( -CaseWidth / 2 + BossInset )"
equation "d1071 = CaseHeight - 8 mm"
equation "d1072 = InsertRadius"
equation "d1073 = InsertDepth"
equation "d1075 = CaseDepth - Cover - InsertDepth"
equation "d1077 = -( -CaseWidth / 2 + BossInset )"
equation "d1078 = CaseHeight - 8 mm"
equation "d1080 = InsertDepth"
equation "d1082 = CaseDepth - 5.8 mm"
equation "d1084 = -( -CaseWidth / 2 + BossInset )"
equation "d1085 = CaseHeight - 8 mm"
equation "d1089 = CaseDepth - 1.8 mm"
equation "d1091 = -( -CaseWidth / 2 + BossInset )"
equation "d1092 = CaseHeight - 8 mm"
equation "d1096 = CaseDepth - 1.8 mm"
equation "d1098 = CaseWidth / 2 - BossInset"
equation "d1103 = CaseDepth - Cover - InsertDepth"
equation "d1105 = CaseWidth / 2 - BossInset"
equation "d1107 = InsertRadius"
equation "d1108 = InsertDepth"
equation "d1110 = CaseDepth - Cover - InsertDepth"
equation "d1112 = CaseWidth / 2 - BossInset"
equation "d1115 = InsertDepth"
equation "d1117 = CaseDepth - 5.8 mm"
equation "d1119 = CaseWidth / 2 - BossInset"
equation "d1124 = CaseDepth - 1.8 mm"
equation "d1126 = CaseWidth / 2 - BossInset"
equation "d1131 = CaseDepth - 1.8 mm"
equation "d1133 = CaseWidth / 2 - BossInset"
equation "d1134 = CaseHeight / 2"
equation "d1138 = CaseDepth - Cover - InsertDepth"
equation "d1140 = CaseWidth / 2 - BossInset"
equation "d1141 = CaseHeight / 2"
equation "d1142 = InsertRadius"
equation "d1143 = InsertDepth"
equation "d1145 = CaseDepth - Cover - InsertDepth"
equation "d1147 = CaseWidth / 2 - BossInset"
equation "d1148 = CaseHeight / 2"
equation "d1150 = InsertDepth"
equation "d1152 = CaseDepth - 5.8 mm"
equation "d1154 = CaseWidth / 2 - BossInset"
equation "d1155 = CaseHeight / 2"
equation "d1159 = CaseDepth - 1.8 mm"
equation "d1161 = CaseWidth / 2 - BossInset"
equation "d1162 = CaseHeight / 2"
equation "d1166 = CaseDepth - 1.8 mm"
equation "d1168 = CaseWidth / 2 - BossInset"
equation "d1169 = CaseHeight - 8 mm"
equation "d1173 = CaseDepth - Cover - InsertDepth"
equation "d1175 = CaseWidth / 2 - BossInset"
equation "d1176 = CaseHeight - 8 mm"
equation "d1177 = InsertRadius"
equation "d1178 = InsertDepth"
equation "d1180 = CaseDepth - Cover - InsertDepth"
equation "d1182 = CaseWidth / 2 - BossInset"
equation "d1183 = CaseHeight - 8 mm"
equation "d1185 = InsertDepth"
equation "d1187 = CaseDepth - 5.8 mm"
equation "d1189 = CaseWidth / 2 - BossInset"
equation "d1190 = CaseHeight - 8 mm"
equation "d1194 = CaseDepth - 1.8 mm"
equation "d1196 = CaseWidth / 2 - BossInset"
equation "d1197 = CaseHeight - 8 mm"
named bodies: "Main housing", "Single rear cover", "Sampling chamber body", "Internal chamber lid — gasket groove TBD", "Potted wire seal envelope TBD", "Right exhaust fitting envelope (1)", "Left inlet fitting envelope", "Guition module envelope", "4.3in active screen", "Carrier side rail", "Carrier side rail (1)", "Future PCB envelope — not routed KiCad board", "Lower PCB component allowance", "Upper PCB component allowance", "FMA holder envelope TBD", "18650 — 3400mAh owner confirmed", "18650 — 3400mAh owner confirmed (1)", "RCY BEC disconnect clearance", "USB mounting insert with integral board supports — seal TBD", "USB interior backing flange", "USB daughterboard — layout TBD", "GCT connector envelope TBD", "USB board support ledge", "USB board support ledge (1)", "12 mm button barrel envelope", "Power button bezel envelope", "Button terminal clearance TBD", "Sensor loom route", "Main cable route", "AO2 body diameter29.3 length31.75", "AO2 M16 neck envelope — no final thread", "AO2 connector and cable allowance", "ZE07-CO total envelope", "MD62 body envelope", "MD62 untrimmed lead allowance", "GYBMEP humidity module envelope TBD", "M3 heat-set insert envelope", "M3 screw shaft envelope", "M3 low head envelope", "M3 heat-set insert envelope (1)", "M3 screw shaft envelope (1)", "M3 low head envelope (1)", "M3 heat-set insert envelope (2)", "M3 screw shaft envelope (2)", "M3 low head envelope (2)", "M3 heat-set insert envelope (3)", "M3 screw shaft envelope (3)", "M3 low head envelope (3)", "M3 heat-set insert envelope (4)", "M3 screw shaft envelope (4)", "M3 low head envelope (4)", "M3 heat-set insert envelope (5)", "M3 screw shaft envelope (5)", "M3 low head envelope (5)"
